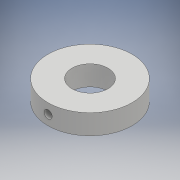
# Autodesk Inventor part: StolLaas
Saved by Autodesk Inventor 2018 (Build 220112000, 112)
## iProperties
Created: 2018-08-31
Part Number: StolLaas
Material: Generic
Document SubType Name: Modeling
Designer: JARVIS
Density: 1 g/cm^3
Appearance: Default
Author: JARVIS
Autodesk Inventor part; units mm, degrees
ref_plane "YZ Plane" through (0, 0, 0) normal (1, 0, 0) x (0, 1, 0)
ref_plane "XZ Plane" through (0, 0, 0) normal (0, 1, 0) x (-1, 0, 0)
ref_plane "XY Plane" through (0, 0, 0) normal (0, 0, 1) x (1, 0, 0)
sketch "Sketch1" plane through (0, 0, 0) normal (0, 0, 1) x (1, 0, 0)
  circle A0 centre (0, 0) radius 4.5
  circle A1 centre (0, 0) radius 10.5
  dimension "d0" = 9
  dimension "d1" = 6
  constraints: 2 centre point, 2 coincident
  measures "d0" diameter of A0
  measures "d1" radial gap between concentric circles of A1 A0
extrude "Extrusion1" add sketch "Sketch1" along normal mid plane 5
sketch "Sketch2" plane through (0, 0, 0) normal (0, 1, 0) x (-1, 0, 0)
  circle A0 centre (0, 0) radius 1
  dimension "d4" = 2
  constraints: 1 centre point, 1 coincident
  measures "d4" diameter of A0
extrude "Extrusion2" cut sketch "Sketch2" against normal through all
body "Solid1"
